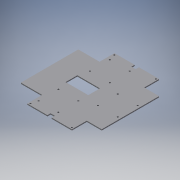
# Autodesk Inventor part: Part37
Saved by Autodesk Inventor 2016 (Build 200138000, 138)
## iProperties
Created: 2015-11-06
Part Number: Part37
Material: Generic
Document SubType Name: Modeling
Designer: Jufo
Density: 1 g/cm^3
Appearance: Default
Author: Jufo
Autodesk Inventor part; units mm, degrees
ref_plane "YZ Plane" through (0, 0, 0) normal (1, 0, 0) x (0, 1, 0)
ref_plane "XZ Plane" through (0, 0, 0) normal (0, 1, 0) x (-1, 0, 0)
ref_plane "XY Plane" through (0, 0, 0) normal (0, 0, 1) x (1, 0, 0)
sketch "Sketch3" plane through (0, 0, 0) normal (0, 1, 0) x (-1, 0, 0)
  line L0 (-63.7605, -81.8282) -> (-41.7605, -81.8282)
  line L1 (-41.7605, -81.8282) -> (-69.7605, -81.8282)
  line L2 (-41.7605, -81.8282) -> (-41.7605, -109.8282)
  line L3 (-41.7605, -81.8282) -> (-41.7605, -109.8282)
  line L4 (-41.7605, -109.8282) -> (-3.7605, -109.8282)
  line L5 (-3.7605, -109.8282) -> (-3.7605, -103.8282)
  line L6 (-3.7605, -109.8282) -> (-3.7605, -103.8282)
  line L7 (-3.7605, -103.8282) -> (4.2395, -103.8282)
  line L8 (4.2395, -103.8282) -> (4.2395, -109.8282)
  line L9 (4.2395, -109.8282) -> (42.2395, -109.8282)
  line L10 (42.2395, -109.8282) -> (42.2395, -81.8282)
  line L11 (42.2395, -109.8282) -> (42.2395, -81.8282)
  line L12 (42.2395, -81.8282) -> (82.2395, -81.8282)
  line L13 (82.2395, -81.8282) -> (82.2395, 26.1718)
  line L14 (42.2395, 26.1718) -> (66.2395, 26.1718)
  line L15 (82.2395, 26.1718) -> (42.2395, 26.1718)
  line L16 (42.2395, 26.1718) -> (42.2395, 54.1718)
  line L17 (42.2395, 54.1718) -> (4.2395, 54.1718)
  line L18 (4.2395, 48.1718) -> (-3.7605, 48.1718)
  line L19 (-3.7605, 48.1718) -> (-3.7605, 54.1718)
  line L20 (4.2395, 48.1718) -> (4.2395, 54.1718)
  line L21 (4.2395, 54.1718) -> (4.2395, 48.1718)
  line L22 (-3.7605, 54.1718) -> (-41.7605, 54.1718)
  line L23 (-41.7605, 54.1718) -> (-41.7605, 26.1718)
  line L24 (-41.7605, 54.1718) -> (-41.7605, 26.1718)
  line L25 (-41.7605, 26.1718) -> (-69.7605, 26.1718)
  line L26 (-69.7605, 26.1718) -> (-69.7605, -81.8282)
  point P0 (0, 0)
  dimension "d1" = 108
  dimension "d2" = 108
  dimension "d3" = 164
  dimension "d4" = 164
  dimension "d6" = 28
  dimension "d7" = 28
  dimension "d11" = 28
  dimension "d12" = 38
  dimension "d13" = 38
  dimension "d14" = 38
  dimension "d15" = 38
  dimension "d16" = 40
  dimension "d18" = 8
  dimension "d19" = 8
  dimension "d21" = 28
  constraints: 54 end point, 9 perpendicular, 6 collinear, 3 horizontal
  measures "d1" distance of L25.end L1.end
  measures "d2" distance of L12.end L13.end
  measures "d3" distance of L22.end L2.end
  measures "d4" distance of L9.end L16.end
  measures "d6" distance of L9.end L10.end
  measures "d7" distance of L0.end L2.end
  measures "d11" distance of L14.start L16.end
  measures "d12" distance between parallel lines of L16 L20
  measures "d13" distance between parallel lines of L23 L19
  measures "d14" distance from line of L7.end L10
  measures "d15" distance from line of L2 L5.end
  measures "d16" distance of L13.end L14.start
  measures "d18" distance of L18.start L18.end
  measures "d19" distance of L5.end L7.end
  measures "d21" distance of L0.end L1.end
extrude "Extrusion1" add sketch "Sketch3" along normal blind 2
sketch "Sketch9" plane through (0, 2, 0) normal (0, 1, 0) x (1, 0, 0)
  circle A0 centre (38.7605, 106.8282) radius 1.5
  line L0 (41.7605, 109.8282) -> (3.7605, 109.8282) projected
  line L1 (41.7605, 81.8282) -> (41.7605, 109.8282) projected
  line L2 (69.7605, -26.1718) -> (69.7605, 81.8282) projected
  line L3 (69.7605, 27.8282) -> (-19.2089, 27.8282)
  line L4 (-0.2395, 109.8282) -> (-0.2395, 42.6367)
  circle A1 centre (-39.2395, 106.8282) radius 1.5
  circle A2 centre (38.7605, -51.1718) radius 1.5
  circle A3 centre (-39.2395, -51.1718) radius 1.5
  point P0 (0, 0)
  dimension "d55" = 3
  dimension "d56" = 3
  dimension "d57" = 3
  constraints: 4 centre point, 4 end point, 3 symmetric about line, 1 horizontal, 1 midpoint, 1 point on line, 1 vertical, 3 other
  measures "d55" diameter of A0
  measures "d56" distance from line of L0 A0.centre
  measures "d57" distance from line of L1 A0.centre
extrude "Extrusion4" cut sketch "Sketch9" against normal blind 10
sketch "Sketch10" plane through (0, 2, 0) normal (0, 1, 0) x (1, 0, 0)
  circle A0 centre (-37.2395, -44.1718) radius 1.5
  circle A1 centre (-37.2395, -44.1718) radius 1.5
  circle A2 centre (-37.2395, -6.8718) radius 1.5
  circle A3 centre (-37.2395, -6.8718) radius 1.5
  circle A4 centre (0.0605, -6.8718) radius 1.5
  circle A5 centre (0.0605, -6.8718) radius 1.5
  circle A6 centre (0.0605, -44.1718) radius 1.5
  circle A7 centre (0.0605, -44.1718) radius 1.5
  line L0 (-42.2395, -54.1718) -> (-4.2395, -54.1718) projected
  line L1 (-42.2395, -26.1718) -> (-42.2395, -54.1718) projected
  line L2 (3.7605, -54.1718) -> (41.7605, -54.1718) projected
  circle A8 centre (0.0605, -44.1718) radius 2.5
  circle A9 centre (0.0605, -6.8718) radius 2.5
  circle A10 centre (-37.2395, -6.8718) radius 2.5
  circle A11 centre (-37.2395, -44.1718) radius 2.5
  point P0 (0, 0)
  point P1 (22.3, 43.3)
  dimension "d60" = 37.3
  dimension "d61" = 37.3
  dimension "d62" = 37.3
  dimension "d63" = 37.3
  dimension "d64" = 10
  dimension "d65" = 5
  dimension "d66" = 5
  dimension "d67" = 10
  dimension "d207" = 5
  dimension "d208" = 5
  dimension "d209" = 5
  dimension "d210" = 5
  constraints: 12 centre point, 8 coincident
  measures "d60" distance of A7.centre A5.centre
  measures "d61" distance of A1.centre A7.centre
  measures "d62" distance of A3.centre A5.centre
  measures "d63" distance of A3.centre A1.centre
  measures "d64" distance from line of L0 A1.centre
  measures "d65" distance from line of L1 A0.centre
  measures "d66" distance from line of L1 A2.centre
  measures "d67" distance from line of L2 A6.centre
  measures "d207" diameter of A8
  measures "d208" diameter of A9
  measures "d209" diameter of A10
  measures "d210" diameter of A11
extrude "Extrusion5" add sketch "Sketch10" along normal blind 5
sketch "Sketch11" plane through (0, 2, 0) normal (0, 1, 0) x (1, 0, 0)
  circle A0 centre (-37.2395, 62.5282) radius 1.5
  circle A1 centre (-37.2395, 62.5282) radius 1.5
  circle A2 centre (-37.2395, 99.8282) radius 1.5
  circle A3 centre (-37.2395, 99.8282) radius 1.5
  circle A4 centre (0.0605, 99.8282) radius 1.5
  circle A5 centre (0.0605, 99.8282) radius 1.5
  circle A6 centre (0.0605, 62.5282) radius 1.5
  circle A7 centre (0.0605, 62.5282) radius 1.5
  line L0 (-4.2395, 109.8282) -> (-42.2395, 109.8282) projected
  line L1 (-42.2395, 109.8282) -> (-42.2395, 81.8282) projected
  circle A8 centre (-37.2395, 62.5282) radius 2.5
  circle A9 centre (-37.2395, 99.8282) radius 2.5
  circle A10 centre (0.0605, 62.5282) radius 2.5
  circle A11 centre (0.0605, 99.8282) radius 2.5
  point P0 (0, 0)
  point P1 (22.3, 43.3)
  dimension "d70" = 37.3
  dimension "d71" = 37.3
  dimension "d72" = 37.3
  dimension "d73" = 37.3
  dimension "d74" = 10
  dimension "d75" = 10
  dimension "d105" = 5
  dimension "d106" = 5
  dimension "d203" = 5
  dimension "d204" = 5
  dimension "d205" = 5
  dimension "d206" = 5
  constraints: 12 centre point, 8 coincident
  measures "d70" distance of A7.centre A5.centre
  measures "d71" distance of A1.centre A7.centre
  measures "d72" distance of A3.centre A1.centre
  measures "d73" distance of A3.centre A5.centre
  measures "d74" distance from line of L0 A4.centre
  measures "d75" distance from line of L0 A2.centre
  measures "d105" distance from line of L1 A3.centre
  measures "d106" distance from line of L1 A1.centre
  measures "d203" diameter of A8
  measures "d204" diameter of A9
  measures "d205" diameter of A10
  measures "d206" diameter of A11
extrude "Extrusion6" add sketch "Sketch11" along normal blind 5
sketch "Sketch12" plane through (0, 2, 0) normal (0, 1, 0) x (1, 0, 0)
  circle A0 centre (27.4605, 9.1782) radius 1.5
  circle A1 centre (27.4605, 9.1782) radius 1.5
  circle A2 centre (27.4605, 46.4782) radius 1.5
  circle A3 centre (27.4605, 46.4782) radius 1.5
  circle A4 centre (64.7605, 46.4782) radius 1.5
  circle A5 centre (64.7605, 46.4782) radius 1.5
  circle A6 centre (64.7605, 9.1782) radius 1.5
  circle A7 centre (64.7605, 9.1782) radius 1.5
  line L0 (69.7605, -26.1718) -> (69.7605, 81.8282) projected
  line L1 (41.7605, -26.1718) -> (69.7605, -26.1718) projected
  circle A8 centre (27.4605, 46.4782) radius 2.5
  circle A9 centre (27.4605, 9.1782) radius 2.5
  circle A10 centre (64.7605, 9.1782) radius 2.5
  circle A11 centre (64.7605, 46.4782) radius 2.5
  point P0 (0, 0)
  point P1 (22.3, 43.3)
  dimension "d80" = 37.3
  dimension "d81" = 37.3
  dimension "d82" = 37.3
  dimension "d83" = 37.3
  dimension "d84" = 5
  dimension "d85" = 5
  dimension "d86" = 35.35
  dimension "d87" = 35.35
  dimension "d199" = 5
  dimension "d200" = 5
  dimension "d201" = 5
  dimension "d202" = 5
  constraints: 12 centre point, 8 coincident
  measures "d80" distance of A4.centre A6.centre
  measures "d81" distance of A1.centre A7.centre
  measures "d82" distance of A3.centre A1.centre
  measures "d83" distance of A5.centre A3.centre
  measures "d84" distance from line of L0 A4.centre
  measures "d85" distance from line of L0 A6.centre
  measures "d86" distance from line of L1 A6.centre
  measures "d87" distance from line of L1 A0.centre
  measures "d199" diameter of A8
  measures "d200" diameter of A9
  measures "d201" diameter of A10
  measures "d202" diameter of A11
extrude "Extrusion7" add sketch "Sketch12" along normal blind 5
sketch "Sketch14" plane through (0, 2, 0) normal (0, 1, 0) x (1, 0, 0)
  line L0 (-41.0232, 16.8213) -> (-41.0232, 38.8213)
  line L1 (-41.0232, 38.8213) -> (1.4768, 38.8213)
  line L2 (1.4768, 38.8213) -> (1.4768, 16.8213)
  line L3 (1.4768, 16.8213) -> (-41.0232, 16.8213)
  point P0 (0, 0)
  dimension "d107" = 22
  dimension "d108" = 42.5
  constraints: 8 end point, 3 perpendicular, 1 vertical
  measures "d107" distance of L0.start L0.end
  measures "d108" distance of L0.end L1.end
extrude "Extrusion9" cut sketch "Sketch14" against normal blind 10
sketch "Sketch17" plane through (0, 2, 0) normal (0, 1, 0) x (1, 0, 0)
  line L0 (-18.0232, -2.1787) -> (-3.0232, -2.1787)
  line L1 (-3.0232, -2.1787) -> (-3.0232, 4.8213)
  line L2 (-3.0232, 4.8213) -> (-18.0232, 4.8213)
  line L3 (-18.0232, 4.8213) -> (-18.0232, -2.1787)
  line L4 (1.4768, 38.8213) -> (1.4768, 16.8213) projected
  line L5 (15.4768, 28.3213) -> (22.4768, 28.3213)
  line L6 (22.4768, 28.3213) -> (22.4768, 43.3213)
  line L7 (22.4768, 43.3213) -> (15.4768, 43.3213)
  line L8 (15.4768, 43.3213) -> (15.4768, 28.3213)
  line L9 (-41.0232, 16.8213) -> (1.4768, 16.8213) projected
  line L10 (-34.0232, 50.8213) -> (-19.0232, 50.8213)
  line L11 (-19.0232, 50.8213) -> (-19.0232, 57.8213)
  line L12 (-19.0232, 57.8213) -> (-34.0232, 57.8213)
  line L13 (-34.0232, 57.8213) -> (-34.0232, 50.8213)
  line L14 (1.4768, 38.8213) -> (-41.0232, 38.8213) projected
  line L15 (-41.0232, 16.8213) -> (-41.0232, 38.8213) projected
  point P0 (0, 0)
  dimension "d148" = 15
  dimension "d149" = 7
  dimension "d150" = 4.5
  dimension "d151" = 7
  dimension "d152" = 15
  dimension "d153" = 12
  dimension "d154" = 14
  dimension "d155" = 15
  dimension "d156" = 7
  dimension "d157" = 12
  dimension "d158" = 7
  dimension "d159" = 10.5
  constraints: 24 end point, 6 parallel, 3 horizontal, 3 perpendicular
  measures "d148" distance of L2.end L1.end
  measures "d149" distance of L1.end L0.end
  measures "d150" distance between parallel lines of L4 L1
  measures "d151" distance of L7.end L6.end
  measures "d152" distance of L6.end L5.end
  measures "d153" distance between parallel lines of L9 L2
  measures "d154" distance between parallel lines of L4 L8
  measures "d155" distance of L12.end L11.end
  measures "d156" distance of L11.end L10.end
  measures "d157" distance between parallel lines of L14 L10
  measures "d158" distance between parallel lines of L15 L13
  measures "d159" distance between parallel lines of L5 L14
extrude "Extrusion12" cut sketch "Sketch17" against normal blind 10 contours L3 L2 L1 L0 | L8 L7 L6 L5 | L13 L12 L11 L10
sketch "Sketch18" plane through (0, 2, 0) normal (0, 1, 0) x (1, 0, 0)
  line L0 (3.4184, -22.7605) -> (10.4184, -22.7605)
  line L1 (10.4184, -22.7605) -> (10.4184, -12.7605)
  line L2 (10.4184, -12.7605) -> (3.4184, -12.7605)
  line L3 (3.4184, -12.7605) -> (3.4184, -22.7605)
  line L4 (3.4184, 68.5282) -> (10.4184, 68.5282)
  line L5 (10.4184, 68.5282) -> (10.4184, 78.5282)
  line L6 (10.4184, 78.5282) -> (3.4184, 78.5282)
  line L7 (3.4184, 78.5282) -> (3.4184, 68.5282)
  line L8 (-47.2883, 68.5282) -> (-40.2883, 68.5282)
  line L9 (-40.2883, 68.5282) -> (-40.2883, 78.5282)
  line L10 (-40.2883, 78.5282) -> (-47.2883, 78.5282)
  line L11 (-47.2883, 78.5282) -> (-47.2883, 68.5282)
  line L12 (-47.2883, -22.9718) -> (-40.2883, -22.9718)
  line L13 (-40.2883, -22.9718) -> (-40.2883, -12.9718)
  line L14 (-40.2883, -12.9718) -> (-47.2883, -12.9718)
  line L15 (-47.2883, -12.9718) -> (-47.2883, -22.9718)
  line L16 (-82.2395, -26.1718) -> (-42.2395, -26.1718) projected
  line L17 (-42.2395, 81.8282) -> (-82.2395, 81.8282) projected
  line L18 (33.2697, 6.0583) -> (43.2697, 6.0583)
  line L19 (43.2697, 6.0583) -> (43.2697, -0.9417)
  line L20 (43.2697, -0.9417) -> (33.2697, -0.9417)
  line L21 (33.2697, -0.9417) -> (33.2697, 6.0583)
  line L22 (33.2697, 49.5137) -> (43.2697, 49.5137)
  line L23 (43.2697, 49.5137) -> (43.2697, 56.5137)
  line L24 (43.2697, 56.5137) -> (33.2697, 56.5137)
  line L25 (33.2697, 56.5137) -> (33.2697, 49.5137)
  point P0 (0, 0)
  dimension "d162" = 7
  dimension "d163" = 10
  dimension "d164" = 7
  dimension "d165" = 10
  dimension "d166" = 7
  dimension "d167" = 10
  dimension "d168" = 10
  dimension "d169" = 3.2
  dimension "d170" = 3.3
  dimension "d171" = 10
  dimension "d172" = 7
  dimension "d173" = 10
  dimension "d174" = 7
  constraints: 48 end point, 12 parallel, 6 horizontal, 6 perpendicular, 5 point on line
  measures "d162" distance of L2.end L1.end
  measures "d163" distance of L1.end L0.end
  measures "d164" distance of L6.end L5.end
  measures "d165" distance of L5.end L4.end
  measures "d166" distance of L10.end L9.end
  measures "d167" distance of L9.end L8.end
  measures "d168" distance of L13.end L12.end
  measures "d169" distance between parallel lines of L12 L16
  measures "d170" distance between parallel lines of L17 L10
  measures "d171" distance of L19.end L20.end
  measures "d172" distance of L18.end L19.end
  measures "d173" distance of L24.end L23.end
  measures "d174" distance of L23.end L22.end
extrude "Extrusion13" cut sketch "Sketch18" against normal blind 10
sketch "Sketch19" plane through (0, 2, 0) normal (0, 1, 0) x (1, 0, 0)
  circle A0 centre (58.2605, -23.6718) radius 1.5
  circle A1 centre (58.2605, -23.6718) radius 1.5
  circle A2 centre (28.4605, -8.4718) radius 1.5
  circle A3 centre (28.4605, -8.4718) radius 1.5
  line L0 (69.7605, -26.1718) -> (69.7605, 81.8282) projected
  line L1 (41.7605, -26.1718) -> (69.7605, -26.1718) projected
  circle A4 centre (58.2605, 64.1282) radius 1.5
  circle A5 centre (58.2605, 64.1282) radius 1.5
  circle A6 centre (28.4605, 79.3282) radius 1.5
  circle A7 centre (28.4605, 79.3282) radius 1.5
  line L2 (69.7605, 81.8282) -> (41.7605, 81.8282) projected
  circle A8 centre (-62.2395, 26.8282) radius 1.5
  circle A9 centre (-47.0395, 56.6282) radius 1.5
  line L3 (-82.2395, 81.8282) -> (-82.2395, -26.1718) projected
  line L4 (-82.2395, -26.1718) -> (-42.2395, -26.1718) projected
  circle A10 centre (-62.2395, 26.8282) radius 2.5
  circle A11 centre (-47.0395, 56.6282) radius 2.5
  circle A12 centre (28.4605, 79.3282) radius 2.5
  circle A13 centre (58.2605, 64.1282) radius 2.5
  circle A14 centre (28.4605, -8.4718) radius 2.5
  circle A15 centre (58.2605, -23.6718) radius 2.5
  point P0 (0, 0)
  point P1 (0, 0)
  point P2 (0, 0)
  dimension "d177" = 15.2
  dimension "d178" = 29.8
  dimension "d179" = 11.5
  dimension "d180" = 2.5
  dimension "d181" = 15.2
  dimension "d182" = 29.8
  dimension "d183" = 2.5
  dimension "d184" = 11.5
  dimension "d185" = 3
  dimension "d186" = 3
  dimension "d187" = 29.8
  dimension "d188" = 15.2
  dimension "d189" = 20
  dimension "d190" = 53
  dimension "d191" = 5
  dimension "d192" = 5
  dimension "d193" = 5
  dimension "d194" = 5
  dimension "d195" = 5
  dimension "d196" = 5
  constraints: 16 centre point, 10 coincident
  measures "d177" vertical distance of A3.centre A1.centre
  measures "d178" horizontal distance of A1.centre A3.centre
  measures "d179" distance from line of L0 A0.centre
  measures "d180" distance from line of L1 A0.centre
  measures "d181" vertical distance of A7.centre A4.centre
  measures "d182" horizontal distance of A4.centre A7.centre
  measures "d183" distance from line of L2 A7.centre
  measures "d184" distance from line of L0 A5.centre
  measures "d185" diameter of A8
  measures "d186" diameter of A9
  measures "d187" vertical distance of A8.centre A9.centre
  measures "d188" horizontal distance of A8.centre A9.centre
  measures "d189" distance from line of L3 A8.centre
  measures "d190" distance from line of L4 A8.centre
  measures "d191" diameter of A10
  measures "d192" diameter of A11
  measures "d193" diameter of A12
  measures "d194" diameter of A13
  measures "d195" diameter of A14
  measures "d196" diameter of A15
extrude "Extrusion14" add sketch "Sketch19" along normal blind 5
equation "\"d7\" = d6"
equation "\"d12\" = d13"
equation "\"d14\" = d13"
equation "\"d15\" = d13"
equation "\"d66\" = d65"
equation "\"d67\" = d64"
equation "\"d75\" = d74"
equation "\"d106\" = d105"
equation "\"d85\" = d84"
equation "\"d87\" = d86"
body "Solid1"
